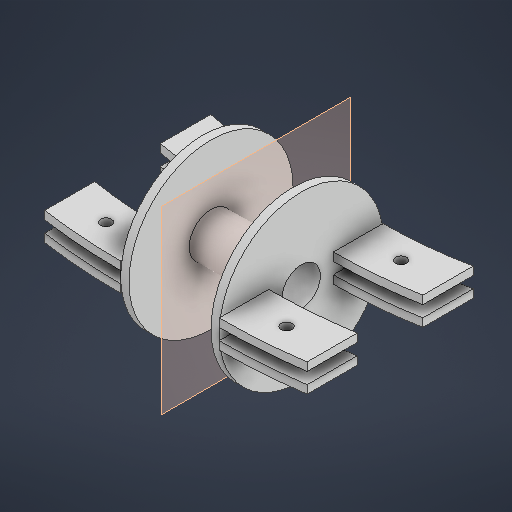
# Autodesk Inventor part: Verbindungsstück
Saved by Autodesk Inventor 2026.1 (Build 301233000, 233)
## iProperties
Created: 2026-01-03
Part Number: Verbindungsstück
Material: Generisch
Document SubType Name: Modeling
Designer: rebsa
Density: 1 g/cm^3
Appearance: Vorgabe
Author: rebsa
Autodesk Inventor part; units mm, degrees
ref_plane "YZ Plane" through (0, 0, 0) normal (1, 0, 0) x (0, 1, 0)
ref_plane "XZ Plane" through (0, 0, 0) normal (0, 1, 0) x (-1, 0, 0)
ref_plane "XY Plane" through (0, 0, 0) normal (0, 0, 1) x (1, 0, 0)
sketch "Skizze1" plane through (0, 0, 0) normal (1, 0, 0) x (0, 1, 0)
  circle A0 centre (0, 0) radius 30
  dimension "d0" = 60
  constraints: 1 centre point, 1 coincident
  measures "d0" diameter of A0
extrude "Extrusion1" add sketch "Skizze1" along normal blind 36
sketch "Skizze2" plane through (0, 0, 0) normal (0, 0, 1) x (1, 0, 0)
  line L0 (0, 30) -> (36, 30) projected
  line L1 (0, -30) -> (36, -30) projected
  line L2 (0, -30) -> (0, 30) projected
  line L3 (36, -30) -> (36, 30) projected
  line L4 (3, 30) -> (33, 30)
  line L5 (33, 30) -> (33, -30)
  line L6 (33, -30) -> (3, -30)
  line L7 (3, -30) -> (3, 30)
  point P0 (0, 0)
  dimension "d3" = 3
  dimension "d4" = 3
  constraints: 8 end point, 2 collinear, 2 parallel, 1 horizontal, 1 perpendicular
  measures "d3" distance between parallel lines of L2 L7
  measures "d4" distance between parallel lines of L3 L5
extrude "Extrusion2" cut sketch "Skizze2" along normal through all both and the other way through all contours L0 L5 L1 L7
sketch "Skizze3" plane through (3, 0, 0) normal (1, 0, 0) x (0, 0, -1)
  circle A0 centre (0, 0) radius 30 projected
  circle A1 centre (0, 0) radius 8
  circle A2 centre (0, 0) radius 7
  point P0 (0, 0)
  dimension "d11" = 16
  dimension "d12" = 14
  constraints: 2 centre point, 2 concentric
  measures "d11" diameter of A1
  measures "d12" diameter of A2
extrude "Extrusion3" add sketch "Skizze3" along normal blind 30 contours A1
sketch "Skizze4" plane through (36, 0, 0) normal (1, 0, 0) x (0, 0, -1)
  circle A0 centre (0, 0) radius 7
  circle A1 centre (0, 0) radius 7 projected
  point P0 (0, 0)
  constraints: 2 concentric, 1 centre point
extrude "Extrusion4" cut sketch "Skizze4" against normal through all
sketch "Skizze9" plane through (0, 0, 0) normal (0, 1, 0) x (-1, 0, 0)
  line L0 (0, 30) -> (-3, 30) projected
  line L1 (0, 30) -> (0, -30) projected
  circle A0 centre (-36, -179.9335) radius 209.9335
  line L2 (0, -208.9659) -> (0, 69.8277) projected
  line L3 (41.5282, 0) -> (-106.5298, 0) projected
  line L4 (-36, 30) -> (-36, -30) projected
  line L5 (-33, 30) -> (-36, 30) projected
  circle A1 centre (-36, -179.9335) radius 191.832
  circle A2 centre (-36, -179.9335) radius 168.168
  circle A3 centre (-36, -179.9335) radius 150.0665
  line L6 (-66, -32.8962) -> (-66, 27.8454)
  point P0 (0, 0)
  point P1 (-66, 9.5382)
  point P2 (-36, 11.8985)
  point P3 (-66, -14.463)
  point P4 (-36, -29.867)
  point P5 (-36, -11.7655)
  dimension "d25" = 300.133
  dimension "d21" = 36
  dimension "d22" = 419.867
  dimension "d23" = 383.664
  dimension "d24" = 336.336
  dimension "d26" = 30
  constraints: 3 centre point, 2 concentric, 2 end point, 2 point on circle, 1 parallel, 1 perpendicular, 4 other
  measures "d21" distance from line of L2 A0.centre
  measures "d22" diameter of A0
  measures "d23" diameter of A1
  measures "d24" diameter of A2
  measures "d26" distance between parallel lines of L4 L6
extrude "Extrusion6" add sketch "Skizze9" along normal mid plane 10.2 contours L4 A1 L6 A0 | L4 A3 L6 A2
sketch "Skizze10" plane through (0, 0, 0) normal (0, 0, 1) x (1, 0, 0)
  line L0 (36, 5.1) -> (36, 5.1) projected
  line L1 (36, 2.8218) -> (36, 5.1) projected
  line L2 (36, -2.8218) -> (36, 2.8218) projected
  line L3 (36, -5.1) -> (36, -2.8218) projected
  line L4 (36, -5.1) -> (36, -5.1) projected
  line L5 (36, 0) -> (36, -5.1) projected
  line L6 (36, 5.1) -> (36, 0) projected
  line L7 (33, -30) -> (33, 30) projected
  line L8 (36, -5.1) -> (36, 0) projected
  line L9 (36, 0) -> (36, 5.1) projected
  line L10 (66, -5.1) -> (66, 5.1) projected
  line L11 (36, 2.1) -> (66, 2.1)
  line L12 (66, 2.1) -> (66, -2.1)
  line L13 (66, -2.1) -> (36, -2.1)
  line L14 (36, -2.1) -> (36, 2.1)
  line L15 (36, -5.1) -> (66, -5.1) projected
  line L16 (36, 5.1) -> (66, 5.1) projected
  point P0 (0, 0)
  point P1 (36, -3.1)
  point P2 (36, 3.1)
  dimension "d29" = 3
  dimension "d45" = 3
  constraints: 8 end point, 2 collinear, 2 parallel, 1 horizontal, 1 perpendicular
  measures "d29" distance between parallel lines of L15 L13
  measures "d45" distance between parallel lines of L16 L11
extrude "Extrusion8" cut sketch "Skizze10" along normal through all both and the other way through all contours L11 L10 L13 L2
sketch "Skizze11" plane through (0, 5.1, 0) normal (0, 1, 0) x (1, 0, 0)
  circle A0 centre (36, 179.9335) radius 159.1175
  line L0 (-245.2362, 0) -> (317.2362, 0) projected
  line L1 (0, 462.9798) -> (0, -112.1633) projected
  line L2 (36, -29.5633) -> (36, 29.5633) projected
  arc A1 (36, 29.867) -> (66, 32.8962) centre (36, 179.9335) ccw projected
  circle A2 centre (36, 179.9335) radius 200.883
  point P0 (0, 0)
  point P1 (51, 21.5246)
  point P2 (51, -20.3887)
  dimension "d34" = 318.235
  dimension "d36" = 401.766
  dimension "d35" = 15
  dimension "d37" = 15
  constraints: 7 other
  measures "d35" distance from line of L2 point (51, 21.525)
  measures "d37" distance from line of L2 point (51, -20.389)
hole "Bohrung1" at (51, 5.1, -21.5246) at (51, 5.1, 20.3887) direction (0, -1, 0) diameter 4 depth 50 tip angle 118
ref_plane "Arbeitsebene1" through (18, 0, 0) normal (1, 0, 0) x (0, 0, -1)
mirror "Spiegeln1" about plane through (18, 0, 0) normal (1, 0, 0) of "Extrusion6", "Bohrung1", "Extrusion8"
